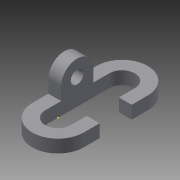
# Autodesk Inventor part: 3-2
Saved by Autodesk Inventor 2015 (Build 190159000, 159)
## iProperties
Created: 2015-09-09
Part Number: 3-2
Material: Generic
Document SubType Name: Modeling
Designer: Brandon
Density: 1 g/cm^3
Appearance: Default
Author: Brandon
Autodesk Inventor part; units mm, degrees
ref_plane "YZ Plane" through (0, 0, 0) normal (1, 0, 0) x (0, 1, 0)
ref_plane "XZ Plane" through (0, 0, 0) normal (0, 1, 0) x (-1, 0, 0)
ref_plane "XY Plane" through (0, 0, 0) normal (0, 0, 1) x (1, 0, 0)
sketch "Sketch1" plane through (0, 0, 0) normal (0, 1, 0) x (-1, 0, 0)
  circle A0 centre (0, 0) radius 25.4
  circle A1 centre (0, -63.5) radius 25.4
  line L0 (25.4, 0) -> (-25.4, 0)
  line L1 (-25.4, 0) -> (-25.4, -63.5)
  line L2 (-25.4, -63.5) -> (25.4, -63.5)
  line L3 (25.4, -63.5) -> (25.4, 0)
  dimension "d0" = 50.8
  dimension "d1" = 50.8
  dimension "d2" = 63.5
  constraints: 8 end point, 2 horizontal alignment, 2 parallel, 1 coincident, 1 horizontal, 1 perpendicular, 4 other
  measures "d2" distance of point (0, -63.5) point (0, 0)
extrude "Extrusion1" add sketch "Sketch1" along normal blind 12.7
sketch "Sketch2" plane through (0, 12.7, 0) normal (0, 1, 0) x (1, 0, 0)
  point P0 (0, 0)
sketch "Sketch3" plane through (0, 12.7, 0) normal (0, 1, 0) x (1, 0, 0)
  point P0 (0, 0)
sketch "Sketch4" plane through (0, 12.7, 0) normal (0, 1, 0) x (1, 0, 0)
  circle A0 centre (0, 0) radius 12.7
  arc A1 (-25.4, 0) -> (25.4, 0) centre (0, 0) ccw projected
  line L0 (0, 0) -> (0, 63.5)
  circle A2 centre (0, 63.5) radius 12.7
  arc A3 (25.4, 63.5) -> (-25.4, 63.5) centre (0, 63.5) ccw projected
  line L1 (-12.7, 0) -> (12.7, 0)
  line L2 (12.7, 0) -> (12.7, 63.5)
  line L3 (12.7, 63.5) -> (-12.7, 63.5)
  line L4 (-12.7, 63.5) -> (-12.7, 0)
  dimension "d5" = 12.7
  dimension "d6" = 63.5
  dimension "d7" = 12.7
  constraints: 10 end point, 2 coincident, 2 horizontal alignment, 2 parallel, 1 horizontal, 1 perpendicular, 1 vertical, 4 other
  measures "d6" distance of L0.start L0.end
extrude "Extrusion2" cut sketch "Sketch4" against normal through all
sketch "Sketch5" plane through (25.4, 0, 0) normal (1, 0, 0) x (0, 0, -1)
  line L0 (0, 0) -> (15.875, 0)
  line L1 (63.5, 0) -> (0, 0) projected
  line L2 (15.875, 0) -> (15.875, 12.7)
  line L3 (0, 12.7) -> (63.5, 12.7) projected
  line L4 (15.875, 12.7) -> (47.625, 12.7)
  line L5 (47.625, 12.7) -> (47.625, 0)
  dimension "d10" = 15.875
  dimension "d11" = 31.75
  constraints: 8 end point, 4 point on line, 1 perpendicular, 1 vertical
  measures "d10" distance of L0.start L0.end
  measures "d11" distance of L2.end L4.end
extrude "Extrusion3" cut sketch "Sketch5" against normal up to next
sketch "Sketch6" plane through (-25.4, 0, -63.5) normal (-1, 0, 0) x (0, 0, 1)
  line L0 (63.5, 12.7) -> (47.625, 12.7)
  line L1 (63.5, 12.7) -> (0, 12.7) projected
  line L2 (47.625, 12.7) -> (47.625, 25.4)
  line L3 (47.625, 25.4) -> (15.875, 25.4)
  line L4 (15.875, 25.4) -> (15.875, 12.7)
  point P0 (63.5, 0)
  dimension "d14" = 15.875
  dimension "d15" = 12.7
  dimension "d16" = 31.75
  constraints: 8 end point, 3 perpendicular, 2 point on line
  measures "d14" distance of L0.start L0.end
  measures "d15" distance of L0.end L2.end
  measures "d16" distance of L2.end L3.end
extrude "Extrusion4" add sketch "Sketch6" against normal blind 12.7
sketch "Sketch7" plane through (-25.4, 0, -63.5) normal (-1, 0, 0) x (0, 0, 1)
  line L0 (47.625, 25.4) -> (15.875, 25.4) projected
  circle A0 centre (31.75, 25.4) radius 15.875
  point P0 (63.5, 0)
  constraints: 1 horizontal alignment, 1 midpoint, 2 other
extrude "Extrusion5" add sketch "Sketch7" against normal blind 12.7
sketch "Sketch8" plane through (-12.7, 0, 0) normal (1, 0, 0) x (0, 0, -1)
  circle A0 centre (31.75, 25.4) radius 6.35
  line L0 (63.5, 0) -> (0, 0) projected
  line L1 (47.625, 25.4) -> (47.625, 12.7)
  arc A1 (47.625, 25.4) -> (15.875, 25.4) centre (31.75, 25.4) ccw projected
  dimension "d21" = 12.7
  dimension "d22" = 25.4
  dimension "d23" = 15.875
  constraints: 2 end point, 1 centre point, 1 tangent, 1 vertical
  measures "d21" diameter of A0
  measures "d22" distance from line of L0 A0.centre
  measures "d23" distance of L1.start A0.centre
extrude "Extrusion6" cut sketch "Sketch8" against normal through all
body "Solid1"
